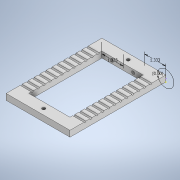
# Autodesk Inventor part: side-A
Saved by Autodesk Inventor 2020 (Build 240168000, 168)
## iProperties
Created: 2020-01-30
Part Number: side-A
Material: Generic
Document SubType Name: Modeling
Designer: pab2
Density: 1 g/cm^3
Appearance: Default
Author: pab2
Autodesk Inventor part; units mm, degrees
ref_plane "YZ Plane" through (0, 0, 0) normal (1, 0, 0) x (0, 1, 0)
ref_plane "XZ Plane" through (0, 0, 0) normal (0, 1, 0) x (-1, 0, 0)
ref_plane "XY Plane" through (0, 0, 0) normal (0, 0, 1) x (1, 0, 0)
sketch "Sketch1" plane through (0, 0, 0) normal (0, 1, 0) x (-1, 0, 0)
  line L0 (0, 0) -> (101.6, 0)
  line L1 (101.6, 0) -> (101.6, -152.4)
  line L2 (101.6, -152.4) -> (0, -152.4)
  line L3 (0, -152.4) -> (0, 0)
  dimension "d0" = 101.6
  dimension "d1" = 152.4
  constraints: 8 end point, 2 parallel, 1 horizontal, 1 perpendicular
  measures "d0" distance of L1.end L2.end
  measures "d1" distance of L0.end L1.end
extrude "Extrusion1" add sketch "Sketch1" along normal blind 9.525
sketch "Sketch2" plane through (0, 9.525, 0) normal (0, 1, 0) x (1, 0, 0)
  line L0 (-101.6, 0) -> (0, 0) projected
  line L1 (0, 0) -> (-17.9605, 17.9605)
  line L2 (0, 0) -> (25.4, 0) construction
  line L3 (-101.6, 152.4) -> (-101.6, 0) projected
  line L4 (-101.6, 152.4) -> (-83.6395, 134.4395)
  line L5 (-17.9605, 17.9605) -> (-83.6395, 17.9605)
  line L6 (-83.6395, 17.9605) -> (-83.6395, 134.4395)
  line L7 (-83.6395, 134.4395) -> (-17.9605, 134.4395)
  line L8 (-17.9605, 134.4395) -> (-17.9605, 17.9605)
  dimension "d4" = 25.4
  dimension "d5" = 135
  dimension "d6" = 25.4
  constraints: 14 end point, 2 horizontal, 2 parallel, 1 equal length, 1 perpendicular
  measures "d4" distance of L0.end L1.end
  measures "d5" angle of L2 L1
  measures "d6" distance of L3.start L4.end
extrude "Extrusion2" cut sketch "Sketch2" against normal blind 9.525 contours L5 L6 L7 L8
sketch "Sketch3" plane through (0, 0, 0) normal (1, 0, 0) x (0, 0, -1)
  line L0 (0, 9.525) -> (152.4, 9.525) projected
  line L1 (0, 10.079) -> (25.4, 10.079) construction
  line L2 (0, 0) -> (0, 9.525) projected
  line L3 (0, 9.525) -> (23.8125, 9.525)
  line L4 (134.4395, 9.525) -> (17.9605, 9.525) projected
  circle A0 centre (23.8125, 9.525) radius 1.5875
  circle A1 centre (33.3375, 9.525) radius 1.5875
  circle A2 centre (42.8625, 9.525) radius 1.5875
  circle A3 centre (52.3875, 9.525) radius 1.5875
  circle A4 centre (61.9125, 9.525) radius 1.5875
  circle A5 centre (71.4375, 9.525) radius 1.5875
  circle A6 centre (80.9625, 9.525) radius 1.5875
  circle A7 centre (90.4875, 9.525) radius 1.5875
  circle A8 centre (100.0125, 9.525) radius 1.5875
  circle A9 centre (109.5375, 9.525) radius 1.5875
  circle A10 centre (119.0625, 9.525) radius 1.5875
  circle A11 centre (128.5875, 9.525) radius 1.5875
  point P0 (130.175, 9.525)
  point P1 (127, 9.525)
  point P2 (120.65, 9.525)
  point P3 (117.475, 9.525)
  point P4 (101.6, 9.525)
  point P5 (98.425, 9.525)
  point P6 (82.55, 9.525)
  point P7 (79.375, 9.525)
  point P8 (73.025, 9.525)
  point P9 (69.85, 9.525)
  point P10 (63.5, 9.525)
  point P11 (60.325, 9.525)
  point P12 (53.975, 9.525)
  point P13 (50.8, 9.525)
  point P14 (44.45, 9.525)
  point P15 (41.275, 9.525)
  point P16 (34.925, 9.525)
  point P17 (31.75, 9.525)
  point P18 (22.225, 9.525)
  point P19 (25.4, 9.525)
  dimension "d11" = 23.8125
  dimension "d12" = 3.175
  dimension "d15" = 9.525
  constraints: 12 centre point, 11 equal radius, 11 horizontal alignment, 4 end point, 1 coincident, 1 horizontal, 1 point on line, 1 other
  measures "d11" distance of L2.end L3.end
  measures "d12" diameter of A0
  measures "d15" distance of A0.centre A1.centre
extrude "Extrusion3" cut sketch "Sketch3" against normal blind 107.95 contours L0 A0 | L0 A11 | L0 A10 | A9 L0 | L0 A9 | L0 A8 | A7 L0 | L0 A7 | L0 A6 | L0 A5 | L0 A4 | L0 A3 | L0 A2 | L0 A1 picked at (24.8555, 9.3984) picked at (128.9035, 8.9629) picked at (119.4808, 8.612) picked at (100.4308, 8.612) picked at (81.3808, 8.612) picked at (71.8558, 8.612) picked at (61.501, 9.0475) picked at (52.5145, 8.7843) picked at (42.9895, 8.7843) picked at (33.5251, 8.5384)
sketch "Sketch4" plane through (0, 0, -152.4) normal (0, 0, -1) x (-1, 0, 0)
  line L0 (101.6, 0) -> (101.6, 9.525) projected
  line L1 (101.6, 4.7625) -> (67.7418, 4.7625)
  line L2 (0, 4.7625) -> (33.8582, 4.7625)
  line L3 (0, 4.7625) -> (33.8582, 4.7625) construction
  point P0 (0, 0)
  dimension "d22" = 33.8582
  dimension "d23" = 33.8582
  dimension "d24" = 0
  constraints: 6 end point, 3 horizontal, 1 collinear, 1 midpoint
  measures "d22" distance of L1.start L1.end
  measures "d23" distance of L2.start L2.end
  measures "d24" distance between parallel lines of L2 L3
hole "Hole1" at (-67.7418, 4.7625, -152.4) direction (0, 0, 1) diameter 4.9784 depth 25.4 thread size "1/4-20 UNC" class "2B" standard "ANSI Unified Screw Threads"
hole "Hole2" at (-33.8582, 4.7625, -152.4) direction (0, 0, 1) diameter 4.9784 depth 25.4 thread size "1/4-20 UNC" class "2B" standard "ANSI Unified Screw Threads"
sketch "Sketch5" plane through (0, 9.525, 0) normal (0, 1, 0) x (1, 0, 0)
  line L0 (-101.6, 0) -> (0, 0) projected
  line L1 (-50.8, 0) -> (-50.8, 17.9605)
  line L2 (-83.6395, 17.9605) -> (-17.9605, 17.9605) projected
  line L3 (-50.8, 0) -> (-50.8, 8.9803)
  constraints: 4 end point, 3 midpoint
sketch "Sketch6" plane through (0, 9.525, 0) normal (0, 1, 0) x (1, 0, 0)
  line L0 (-17.9605, 134.4395) -> (-83.6395, 134.4395) projected
  line L1 (-50.8, 134.4395) -> (-50.8, 152.4)
  line L2 (0, 152.4) -> (-101.6, 152.4) projected
  line L3 (-50.8, 134.4395) -> (-50.8, 143.4197)
  point P0 (0, 0)
  constraints: 4 end point, 3 midpoint
hole "Hole3" at (-50.8, 9.525, -8.9803) direction (0, -1, 0) diameter 4.9784 depth 25.4 thread size "1/4-20 UNC" class "2B" standard "ANSI Unified Screw Threads"
hole "Hole4" at (-50.8, 9.525, -143.4197) direction (0, -1, 0) diameter 4.9784 depth 25.4 thread size "1/4-20 UNC" class "2B" standard "ANSI Unified Screw Threads"
body "Solid1"
